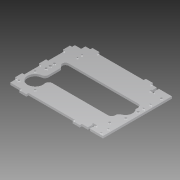
# Autodesk Inventor part: plastic_part_52
Saved by Autodesk Inventor 2013 (Build 170138000, 138)
## iProperties
Shininess: 20.0
Created: 2013-07-01
Part Number: plastic_part_52
Document SubType Name: Modeling
Designer: Noa Izumi
Material: Default
Density: 1 g/cm^3
Density: 0.0
Volumn: 0.0
Area: 0.0
PropertySet Name: Model Information
Control State: 0
Master: False
Checked Out: False
Author: Noa Izumi
Autodesk Inventor part; units mm, degrees
ref_plane "YZ Plane" through (0, 0, 0) normal (1, 0, 0) x (0, 1, 0)
ref_plane "XZ Plane" through (0, 0, 0) normal (0, 1, 0) x (-1, 0, 0)
ref_plane "XY Plane" through (0, 0, 0) normal (0, 0, 1) x (1, 0, 0)
sketch "Sketch1" plane through (0, 0, 0) normal (0, 0, 1) x (1, 0, 0)
  line L0 (0, 0) -> (132, 0)
  line L1 (132, 0) -> (132, 98)
  line L2 (132, 98) -> (0, 98)
  line L3 (0, 98) -> (0, 0)
  line L4 (16, 101) -> (26, 101)
  line L5 (26, 101) -> (26, -3)
  line L6 (26, -3) -> (16, -3)
  line L7 (16, -3) -> (16, 101)
  line L8 (102, 101) -> (92, 101)
  line L9 (92, 101) -> (92, -3)
  line L10 (92, -3) -> (102, -3)
  line L11 (102, -3) -> (102, 101)
  line L12 (0, 88) -> (-3, 88)
  line L13 (-3, 88) -> (-3, 78)
  line L14 (-3, 78) -> (0, 78)
  line L15 (0, 78) -> (0, 88)
  line L16 (0, 10) -> (-3, 10)
  line L17 (-3, 10) -> (-3, 20)
  line L18 (-3, 20) -> (0, 20)
  line L19 (0, 20) -> (0, 10)
  line L20 (0, 54) -> (-3, 54)
  line L21 (-3, 54) -> (-3, 44)
  line L22 (-3, 44) -> (0, 44)
  line L23 (0, 44) -> (0, 54)
  line L24 (0, 98) -> (9, 98)
  line L25 (9, 98) -> (9, 93)
  line L26 (8, 92) -> (0, 92)
  line L27 (0, 92) -> (0, 98)
  arc A0 (8, 92) -> (9, 93) centre (8, 93) ccw
  point P0 (9, 92)
  dimension "d0" = 98
  dimension "d1" = 132
  dimension "d74" = 10
  dimension "d77" = 10
  dimension "d306" = 16
  dimension "d307" = 104
  dimension "d308" = 3
  dimension "d309" = 3
  dimension "d310" = 104
  dimension "d311" = 30
  dimension "d312" = 3
  dimension "d313" = 10
  dimension "d314" = 10
  dimension "d315" = 3
  dimension "d316" = 10
  dimension "d317" = 10
  dimension "d318" = 10
  dimension "d319" = 3
  dimension "d320" = 24
  dimension "d368" = 9
  dimension "d369" = 6
  dimension "d370" = 1
  constraints: 56 end point, 14 parallel, 7 horizontal, 7 perpendicular, 5 point on line, 2 point on circle, 2 tangent, 1 centre point
  measures "d0" distance of L2.end L0.start
  measures "d1" distance of L0.start L0.end
  measures "d74" distance of L5.end L6.end
  measures "d77" distance of L9.end L10.end
  measures "d306" distance between parallel lines of L7 L3
  measures "d307" distance of L6.end L4.start
  measures "d308" distance between parallel lines of L0 L6
  measures "d309" distance between parallel lines of L0 L10
  measures "d310" distance of L8.end L9.end
  measures "d311" distance between parallel lines of L1 L11
  measures "d312" distance of L13.end L14.end
  measures "d313" distance of L12.end L13.end
  measures "d314" distance from line of L12.end L2
  measures "d315" distance of L16.start L16.end
  measures "d316" distance of L16.end L17.end
  measures "d317" distance from line of L0 L16.end
  measures "d318" distance of L20.end L21.end
  measures "d319" distance of L20.start L20.end
  measures "d320" distance between parallel lines of L18 L22
  measures "d368" distance of point (9, 92) L26.end
  measures "d369" distance of L24.end point (9, 92)
  measures "d370" radius of A0
extrude "Extrusion1" add sketch "Sketch1" along normal blind 3 contours L3 L26 A0 L25 L2 L7 L0 | L7 L2 L5 L0 | L0 L5 L6 L7 | L16 L17 L18 L3 | L5 L2 L9 L0 | L7 L4 L5 L2 | L9 L2 L11 L0 | L0 L11 L10 L9 | L22 L21 L20 L3 | L11 L2 L1 L0 | L9 L8 L11 L2 | L14 L13 L12 L3
sketch "Sketch11" plane through (0, 0, 3) normal (0, 0, 1) x (1, 0, 0)
  line L0 (0, 0) -> (0, 98) projected
  line L1 (6, 0) -> (0, 0) projected
  point P0 (15, 20.5)
  dimension "d141" = 20.5
  dimension "d142" = 15
  measures "d141" distance from line of L1 point (15, 20.5)
  measures "d142" distance from line of point (15, 20.5) L0
hole "Hole7" at (15, 20.5, 3) direction (0, 0, -1) diameter 22 end through all
sketch "Sketch12" plane through (0, 0, 3) normal (0, 0, 1) x (1, 0, 0)
  circle A0 centre (15, 20.5) radius 11 projected
  point P0 (3.5, 32)
  point P1 (26.5, 9)
  point P2 (3.5, 9)
  dimension "d152" = 11.5
  dimension "d153" = 11.5
  dimension "d161" = 11.5
  dimension "d162" = 11.5
  dimension "d163" = 11.5
  dimension "d164" = 11.5
  measures "d152" horizontal distance of A0.centre point (3.5, 32)
  measures "d153" horizontal distance of point (26.5, 9) A0.centre
  measures "d161" horizontal distance of point (3.5, 32) A0.centre
  measures "d162" horizontal distance of point (3.5, 9) A0.centre
  measures "d163" horizontal distance of A0.centre point (3.5, 9)
  measures "d164" horizontal distance of A0.centre point (26.5, 9)
hole "Hole8" at (3.5, 32, 3) at (26.5, 9, 3) at (3.5, 9, 3) direction (0, 0, -1) diameter 2.5 end through all
sketch "Sketch20" plane through (0, 0, 3) normal (0, 0, 1) x (1, 0, 0)
  line L0 (132, 0) -> (120, 0) projected
  line L1 (132, 98) -> (132, 0) projected
  line L2 (120, 98) -> (132, 98) projected
  line L3 (125.5, 73.7) -> (128, 73.7)
  line L4 (128, 73.7) -> (128, 72.3)
  line L5 (128, 72.3) -> (125.5, 72.3)
  line L6 (125.5, 72.3) -> (125.5, 73.7)
  line L7 (125.5, 63.7) -> (128, 63.7)
  line L8 (128, 63.7) -> (128, 62.3)
  line L9 (128, 62.3) -> (125.5, 62.3)
  line L10 (125.5, 62.3) -> (125.5, 63.7)
  line L11 (125.5, 13.7) -> (128, 13.7)
  line L12 (128, 13.7) -> (128, 12.3)
  line L13 (128, 12.3) -> (125.5, 12.3)
  line L14 (125.5, 12.3) -> (125.5, 13.7)
  line L15 (125.5, 3.7) -> (128, 3.7)
  line L16 (128, 3.7) -> (128, 2.3)
  line L17 (128, 2.3) -> (125.5, 2.3)
  line L18 (125.5, 2.3) -> (125.5, 3.7)
  dimension "d208" = 1.4
  dimension "d209" = 24.3
  dimension "d210" = 4
  dimension "d211" = 2.5
  dimension "d212" = 1.4
  dimension "d213" = 8.6
  dimension "d214" = 2.5
  dimension "d215" = 1.4
  dimension "d216" = 2.3
  dimension "d217" = 4
  dimension "d218" = 8.6
  dimension "d219" = 1.4
  constraints: 32 end point, 8 parallel, 4 horizontal, 4 perpendicular
  measures "d208" distance of L3.end L4.end
  measures "d209" distance between parallel lines of L2 L3
  measures "d210" distance between parallel lines of L1 L4
  measures "d211" distance of L3.start L3.end
  measures "d212" distance of L7.end L8.end
  measures "d213" distance between parallel lines of L7 L5
  measures "d214" distance of L16.end L17.end
  measures "d215" distance of L15.end L16.end
  measures "d216" distance between parallel lines of L0 L17
  measures "d217" distance between parallel lines of L1 L16
  measures "d218" distance between parallel lines of L15 L13
  measures "d219" distance of L11.end L12.end
extrude "Extrusion10" cut sketch "Sketch20" against normal through all
sketch "Sketch26" plane through (0, 0, 3) normal (0, 0, 1) x (1, 0, 0)
  line L0 (0, 98) -> (6, 98) projected
  line L1 (0, 88) -> (0, 98) projected
  point P0 (17, 85.25)
  point P1 (17, 78.75)
  dimension "d289" = 6.5
  dimension "d290" = 12.75
  dimension "d366" = 17
  measures "d289" distance of point (17, 78.75) point (17, 85.25)
  measures "d290" distance from line of L0 point (17, 85.25)
  measures "d366" distance from line of point (17, 85.25) L1
hole "Hole13" at (17, 85.25, 3) at (17, 78.75, 3) direction (0, 0, -1) diameter 2 end through all
sketch "草圖28" plane through (0, 0, 3) normal (0, 0, 1) x (1, 0, 0)
  line L0 (132, 0) -> (102, 0) projected
  line L1 (132, 98) -> (132, 0) projected
  line L2 (102, 98) -> (132, 98) projected
  line L3 (110.5, 98) -> (113.5, 98)
  line L4 (113.5, 98) -> (113.5, 89)
  line L5 (113.5, 89) -> (110.5, 89)
  line L6 (110.5, 89) -> (110.5, 98)
  line L7 (109.25, 89) -> (114.75, 89)
  line L8 (114.75, 89) -> (114.75, 91.3)
  line L9 (114.75, 91.3) -> (109.25, 91.3)
  line L10 (109.25, 91.3) -> (109.25, 89)
  line L11 (113.5, 9) -> (110.5, 9)
  line L12 (110.5, 9) -> (110.5, 0)
  line L13 (110.5, 0) -> (113.5, 0)
  line L14 (113.5, 0) -> (113.5, 9)
  line L15 (109.25, 9) -> (114.75, 9)
  line L16 (114.75, 9) -> (114.75, 6.7)
  line L17 (114.75, 6.7) -> (109.25, 6.7)
  line L18 (109.25, 6.7) -> (109.25, 9)
  dimension "d321" = 9
  dimension "d323" = 3
  dimension "d324" = 5.5
  dimension "d325" = 2.3
  dimension "d326" = 1.25
  dimension "d327" = 18.5
  dimension "d328" = 18.5
  dimension "d329" = 9
  dimension "d330" = 5.5
  dimension "d331" = 2.3
  dimension "d378" = 1.25
  constraints: 32 end point, 8 parallel, 4 horizontal, 4 perpendicular, 3 point on line
  measures "d321" distance of L5.end L3.start
  measures "d323" distance of L4.end L5.end
  measures "d324" distance of L7.start L7.end
  measures "d325" distance of L7.end L8.end
  measures "d326" distance between parallel lines of L6 L10
  measures "d327" distance between parallel lines of L1 L4
  measures "d328" distance between parallel lines of L1 L14
  measures "d329" distance of L13.end L11.start
  measures "d330" distance of L15.start L15.end
  measures "d331" distance of L15.end L16.end
  measures "d378" distance between parallel lines of L12 L18
extrude "擠出14" cut sketch "草圖28" against normal through all
sketch "草圖29" plane through (0, 0, 3) normal (0, 0, 1) x (1, 0, 0)
  line L0 (26, 98) -> (16, 98) projected
  line L1 (0, 54) -> (0, 78) projected
  point P0 (0, 98)
  point P1 (8, 49)
  dimension "d336" = 8
  dimension "d337" = 49
  measures "d336" distance from line of point (8, 49) L1
  measures "d337" distance from line of point (8, 49) L0
hole "孔14" at (8, 49, 3) direction (0, 0, -1) diameter 3.5 end through all
sketch "草圖30" plane through (0, 0, 3) normal (0, 0, 1) x (1, 0, 0)
  circle A0 centre (8, 49) radius 1.75 projected
  line L0 (132, 0) -> (113.5, 0) projected
  line L1 (132, 98) -> (132, 0) projected
  line L2 (113.5, 98) -> (132, 98) projected
  point P0 (8, 55)
  point P1 (8, 43)
  point P2 (120, 21.5)
  point P3 (126, 38.5)
  point P4 (127, 55)
  point P5 (127, 88)
  dimension "d345" = 6
  dimension "d346" = 6
  dimension "d371" = 21.5
  dimension "d372" = 12
  dimension "d373" = 6
  dimension "d374" = 38.5
  dimension "d375" = 5
  dimension "d376" = 55
  dimension "d377" = 10
  dimension "d381" = 5
  measures "d345" distance of A0.centre point (8, 55)
  measures "d346" distance of A0.centre point (8, 43)
  measures "d371" distance from line of L0 point (120, 21.5)
  measures "d372" distance from line of L1 point (120, 21.5)
  measures "d373" distance from line of L1 point (126, 38.5)
  measures "d374" distance from line of L0 point (126, 38.5)
  measures "d375" distance from line of L1 point (127, 55)
  measures "d376" distance from line of L0 point (127, 55)
  measures "d377" distance from line of point (127, 88) L2
  measures "d381" distance from line of L1 point (127, 88)
hole "孔15" at (8, 55, 3) at (8, 43, 3) at (127, 88, 3) at (127, 55, 3) at (126, 38.5, 3) at (120, 21.5, 3) direction (0, 0, -1) diameter 3 end through all
sketch "草圖31" plane through (0, 0, 3) normal (0, 0, 1) x (1, 0, 0)
  line L0 (26, 98) -> (92, 98) projected
  line L1 (0, 54) -> (0, 78) projected
  line L2 (18, 65) -> (117, 65)
  line L3 (110, 29.25) -> (18, 29.25)
  line L4 (18, 29.25) -> (18, 52.4223)
  arc A0 (18, 65) -> (15.6316, 56.6737) centre (18, 60.5) ccw
  arc A1 (118.3333, 39.5719) -> (122, 56.1414) centre (115, 49) ccw
  line L5 (115, 34.25) -> (115, 34.8579)
  line L6 (122, 60) -> (122, 56.1414)
  arc A2 (18, 52.4223) -> (15.6316, 56.6737) centre (13, 52.4223) ccw
  arc A3 (122, 60) -> (117, 65) centre (117, 60) ccw
  arc A4 (118.3333, 39.5719) -> (115, 34.8579) centre (120, 34.8579) ccw
  arc A5 (110, 29.25) -> (115, 34.25) centre (110, 34.25) ccw
  line L7 (132, 98) -> (132, 0) projected
  point P0 (115, 39)
  point P1 (18, 56)
  point P2 (132, 86.882)
  dimension "d354" = 35.75
  dimension "d356" = 33
  dimension "d358" = 18
  dimension "d359" = 9
  dimension "d360" = 20
  dimension "d362" = 5
  dimension "d379" = 10
  dimension "d380" = 17
  constraints: 14 point on circle, 10 end point, 8 tangent, 6 centre point, 3 equal radius, 3 point on line, 2 parallel, 1 horizontal, 1 perpendicular
  measures "d354" distance between parallel lines of L3 L2
  measures "d356" distance between parallel lines of L0 L2
  measures "d358" distance between parallel lines of L4 L1
  measures "d359" diameter of A0
  measures "d360" diameter of A1
  measures "d362" radius of A2
  measures "d379" distance between parallel lines of L7 L6
  measures "d380" distance from line of L7 A1.centre
extrude "擠出15" cut sketch "草圖31" against normal through all
fillet "圓角9" radius 5 2 edges at (18, 31.083, 1.5) (21.6661, 29.25, 1.5)
